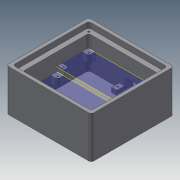
# Autodesk Inventor part: Part1
Saved by Autodesk Inventor 2014 SP1 (Build 180222100, 222)
## iProperties
Created: 2015-04-01
Part Number: Part1
Material: Generic
Document SubType Name: Modeling
Designer: tom
Density: 1 g/cm^3
Appearance: Default
Author: tom
Autodesk Inventor part; units mm, degrees
note: some values were not read from the file. Chosen so that the rebuilt part matches the saved one: sketch regions of "Extrusion8".
ref_plane "YZ Plane" through (0, 0, 0) normal (1, 0, 0) x (0, 1, 0)
ref_plane "XZ Plane" through (0, 0, 0) normal (0, 1, 0) x (-1, 0, 0)
ref_plane "XY Plane" through (0, 0, 0) normal (0, 0, 1) x (1, 0, 0)
sketch "Sketch1" plane through (0, 0, 0) normal (0, 1, 0) x (-1, 0, 0)
  line L0 (80.9542, -63.5193) -> (-4.7708, -63.5193)
  line L1 (-4.7708, -63.5193) -> (-4.7708, 19.0307)
  line L2 (-4.7708, 19.0307) -> (80.9542, 19.0307)
  line L3 (80.9542, 19.0307) -> (80.9542, -63.5193)
  line L4 (-14.7708, -73.5193) -> (90.9542, -73.5193)
  line L5 (90.9542, -73.5193) -> (90.9542, 29.0307)
  line L6 (90.9542, 29.0307) -> (-14.7708, 29.0307)
  line L7 (-14.7708, 29.0307) -> (-14.7708, -73.5193)
  point P0 (0, 0)
  dimension "d0" = 85.725
  dimension "d1" = 82.55
  dimension "d2" = 10
  constraints: 16 end point, 4 parallel, 2 perpendicular, 1 horizontal, 3 other
  measures "d0" distance of L0.start L0.end
  measures "d1" distance of L0.end L1.end
  measures "d2" distance between parallel lines of L3 L5
extrude "Extrusion1" add sketch "Sketch1" along normal blind 5 contours L0 L1 L2 L3 | L7 L6 L5 L4
sketch "Sketch2" plane through (0, 5, 0) normal (0, 1, 0) x (1, 0, 0)
  line L0 (14.7708, 73.5193) -> (-90.9542, 73.5193) projected
  line L1 (-90.9542, 73.5193) -> (-90.9542, -29.0307) projected
  line L2 (-90.9542, -29.0307) -> (14.7708, -29.0307) projected
  line L3 (14.7708, -29.0307) -> (14.7708, 73.5193) projected
  line L4 (-80.9542, 63.5193) -> (4.7708, 63.5193)
  line L5 (4.7708, 63.5193) -> (4.7708, -19.0307)
  line L6 (4.7708, -19.0307) -> (-80.9542, -19.0307)
  line L7 (-80.9542, -19.0307) -> (-80.9542, 63.5193)
  point P0 (0, 0)
  dimension "d5" = 85.725
  dimension "d6" = 82.55
  dimension "d7" = 10
  dimension "d8" = 10
  constraints: 8 end point, 3 perpendicular, 1 parallel
  measures "d5" distance of L4.start L4.end
  measures "d6" distance of L4.end L5.end
  measures "d7" distance between parallel lines of L1 L7
  measures "d8" distance between parallel lines of L0 L4
extrude "Extrusion2" add sketch "Sketch2" along normal blind 40
fillet "Fillet1" radius 3.175 8 edges at (-80.9542, 25, -63.5193) (4.7708, 25, -63.5193) (-80.9542, 25, 19.0307) (4.7708, 25, 19.0307) (-90.9542, 22.5, -73.5193) (14.7708, 22.5, -73.5193) (-90.9542, 22.5, 29.0307) (14.7708, 22.5, 29.0307)
sketch "Sketch3" plane through (11.5958, 0, -73.5193) normal (0, 0, -1) x (-1, 0, 0)
  line L0 (10, 5) -> (89.375, 5) projected
  circle A0 centre (25.875, 8.175) radius 2.3813
  circle A1 centre (35.4, 8.175) radius 2.3812
  circle A2 centre (44.925, 8.175) radius 2.3812
  circle A3 centre (25.875, 17.7) radius 2.3812
  circle A4 centre (44.925, 17.7) radius 2.3812
  line L1 (6.825, 45) -> (6.825, 5) projected
  line L2 (25.875, 20.0813) -> (44.925, 20.0813)
  line L3 (47.3062, 17.7) -> (47.3062, 8.175)
  line L4 (44.925, 5.7938) -> (25.875, 5.7937)
  line L5 (23.4937, 8.175) -> (23.4937, 17.7)
  point P0 (11.5958, 0)
  dimension "d12" = 4.7625
  dimension "d13" = 4.7625
  dimension "d14" = 4.7625
  dimension "d15" = 9.525
  dimension "d16" = 9.525
  dimension "d17" = 3.175
  dimension "d18" = 4.7625
  dimension "d19" = 4.7625
  dimension "d20" = 9.525
  dimension "d21" = 9.525
  dimension "d22" = 19.05
  dimension "d23" = 19.05
  constraints: 8 end point, 8 point on circle, 5 centre point, 5 tangent, 2 perpendicular
  measures "d12" diameter of A0
  measures "d13" diameter of A1
  measures "d14" diameter of A2
  measures "d15" distance of A0.centre A1.centre
  measures "d16" distance of A2.centre A1.centre
  measures "d17" distance from line of L0 A0.centre
  measures "d18" diameter of A3
  measures "d19" diameter of A4
  measures "d20" distance of A0.centre A3.centre
  measures "d21" distance of A4.centre A2.centre
  measures "d22" distance from line of L1 A0.centre
  measures "d23" distance of A4.centre A3.centre
extrude "Extrusion3" cut sketch "Sketch3" against normal blind 10 contours A0 | A1 | A0 L5 A3 L2 A4 L3 A2 L4 | A3 | A2 | A4
sketch "Sketch4" plane through (-77.7792, 5, -63.5193) normal (0, 0, 1) x (1, 0, 0)
  arc A0 (63.5, 0.7937) -> (65.8813, 3.175) centre (63.5, 3.175) ccw projected
  line L0 (63.5, 0.7937) -> (44.45, 0.7938) projected
  arc A1 (42.0688, 3.175) -> (44.45, 0.7938) centre (44.45, 3.175) ccw projected
  line L1 (79.375, 40) -> (79.375, 0) projected
  line L2 (79.375, 0) -> (0, 0) projected
  circle A2 centre (44.45, 3.175) radius 2.3812
  circle A3 centre (63.5, 3.175) radius 2.3813
  circle A4 centre (53.975, 3.175) radius 2.3812
  line L3 (46.8313, 3.175) -> (47.698, 5.5563)
  line L4 (46.8313, 3.175) -> (49.3653, 3.175) construction
  line L5 (51.5938, 3.175) -> (50.727, 5.5563)
  line L6 (51.5938, 3.175) -> (54.1278, 3.175) construction
  line L7 (50.727, 5.5563) -> (47.698, 5.5563)
  line L8 (56.3563, 3.175) -> (57.223, 5.5563)
  line L9 (61.1188, 3.175) -> (60.252, 5.5563)
  line L10 (60.252, 5.5563) -> (57.223, 5.5563)
  line L11 (42.0688, 3.175) -> (41.202, 5.5563)
  line L12 (41.202, 5.5563) -> (34.852, 5.5563)
  line L13 (34.852, 5.5563) -> (34.852, 0)
  line L14 (65.8813, 3.175) -> (66.748, 5.5562)
  line L15 (66.748, 5.5562) -> (73.098, 5.5562)
  line L16 (0, 0) -> (0, 40) projected
  line L17 (73.098, 5.5562) -> (73.098, 0)
  point P0 (77.7792, -5)
  dimension "d26" = 70
  dimension "d27" = 110
  dimension "d28" = 6.35
  dimension "d31" = 6.35
  constraints: 28 end point, 6 parallel, 6 point on circle, 3 centre point, 2 coincident, 2 collinear, 2 equal length, 2 horizontal, 2 perpendicular, 2 point on line
  measures "d26" angle of L4 L3
  measures "d27" angle of L6 L5
  measures "d28" distance of L11.end L12.end
  measures "d31" distance of L14.end L15.end
extrude "Extrusion4" add sketch "Sketch4" along normal blind 9.525 contours A0 L14 L15 L17 L2 L13 L12 L11 A1 L0 | L0 A4 L8 L10 L9 A3 | L0 A2 L3 L7 L5 A4
ref_plane "Work Plane1" through (-40.0917, 29.5, -24.6568) normal (0, -1, 0) x (1, 0, 0)
sketch "Sketch6" plane through (0, 45, 0) normal (0, 1, 0) x (1, 0, 0)
  arc A0 (11.5958, -29.0307) -> (14.7708, -25.8557) centre (11.5958, -25.8557) ccw projected
  line L0 (14.7708, -25.8557) -> (14.7708, 70.3443) projected
  arc A1 (14.7708, 70.3443) -> (11.5958, 73.5193) centre (11.5958, 70.3443) ccw projected
  line L1 (11.5958, 73.5193) -> (-87.7792, 73.5193) projected
  arc A2 (-87.7792, 73.5193) -> (-90.9542, 70.3443) centre (-87.7792, 70.3443) ccw projected
  line L2 (-90.9542, 70.3443) -> (-90.9542, -25.8557) projected
  arc A3 (-90.9542, -25.8557) -> (-87.7792, -29.0307) centre (-87.7792, -25.8557) ccw projected
  line L3 (-87.7792, -29.0307) -> (11.5958, -29.0307) projected
  line L4 (-86.9542, 69.5193) -> (10.7708, 69.5193)
  line L5 (10.7708, 69.5193) -> (10.7708, -25.0307)
  line L6 (10.7708, -25.0307) -> (-86.9542, -25.0307)
  line L7 (-86.9542, -25.0307) -> (-86.9542, 69.5193)
  point P0 (0, 0)
  dimension "d38" = 4
  dimension "d39" = 4
  dimension "d40" = 4
  dimension "d41" = 4
  constraints: 8 end point, 2 parallel, 1 horizontal, 1 perpendicular
  measures "d38" distance between parallel lines of L1 L4
  measures "d39" distance between parallel lines of L2 L7
  measures "d40" distance between parallel lines of L3 L6
  measures "d41" distance between parallel lines of L0 L5
extrude "Extrusion6" add sketch "Sketch6" along normal blind 7
fillet "Fillet2" radius 3.175 4 edges at (10.7708, 48.5, -69.5193) (-86.9542, 48.5, -69.5193) (-86.9542, 48.5, 25.0307) (10.7708, 48.5, 25.0307)
sketch "Sketch7" plane through (0, 45, 0) normal (0, 1, 0) x (1, 0, 0)
  line L0 (7.5958, 69.5193) -> (-83.7792, 69.5193) projected
  line L1 (4.7708, 60.3443) -> (4.7708, -15.8557) projected
  line L2 (1.5958, -19.0307) -> (-77.7792, -19.0307) projected
  line L3 (-80.9542, -15.8557) -> (-80.9542, 60.3443) projected
  arc A0 (-77.7792, 63.5193) -> (-80.9542, 60.3443) centre (-77.7792, 60.3443) ccw projected
  line L4 (-38.0917, 69.5193) -> (-38.0917, -19.0307) construction
  line L5 (-80.9542, 22.2443) -> (4.7708, 22.2443) construction
  line L6 (-77.7792, 60.3443) -> (-82.7289, 65.2941) construction
  circle A1 centre (-82.7289, 65.2941) radius 1.27
  circle A2 centre (6.5456, 65.2941) radius 1.27
  circle A3 centre (-82.7289, -20.8054) radius 1.27
  circle A4 centre (6.5456, -20.8054) radius 1.27
  point P0 (0, 0)
  dimension "d44" = 7
  dimension "d45" = 2.54
  constraints: 6 end point, 4 centre point, 4 midpoint, 3 symmetric about line, 1 coincident, 3 other
  measures "d44" distance of L6.start L6.end
  measures "d45" diameter of A1
extrude "Extrusion7" cut sketch "Sketch7" against normal blind 12.7
sketch "Sketch8" plane through (-40.0917, 29.5, -24.6568) normal (0, -1, 0) x (1, 0, 0)
  circle A0 centre (39.5, -2.5) radius 1 projected
  circle A1 centre (39.5, -33.5) radius 1 projected
  circle A2 centre (-35.5, -2.5) radius 1 projected
  circle A3 centre (-35.5, -33.5) radius 1 projected
  line L0 (-38, 0) -> (42, 0) projected
  line L1 (-38, -36) -> (-38, 0) projected
  line L2 (42, -36) -> (-38, -36) projected
  line L3 (42, 0) -> (42, -36) projected
  arc A4 (39.5, -30.5) -> (36.5, -33.5) centre (39.5, -33.5) ccw
  circle A5 centre (-42.6372, 45.4622) radius 1.27 projected
  circle A6 centre (-42.6372, -40.6372) radius 1.27 projected
  circle A7 centre (46.6372, -40.6372) radius 1.27 projected
  circle A8 centre (46.6372, 45.4622) radius 1.27 projected
  arc A9 (50.8625, 46.5125) -> (47.6875, 49.6875) centre (47.6875, 46.5125) ccw projected
  line L4 (50.8625, 46.5125) -> (50.8625, -41.6875) projected
  arc A10 (47.6875, -44.8625) -> (50.8625, -41.6875) centre (47.6875, -41.6875) ccw projected
  line L5 (47.6875, -44.8625) -> (-43.6875, -44.8625) projected
  arc A11 (-46.8625, -41.6875) -> (-43.6875, -44.8625) centre (-43.6875, -41.6875) ccw projected
  line L6 (-46.8625, -41.6875) -> (-46.8625, 46.5125) projected
  arc A12 (-43.6875, 49.6875) -> (-46.8625, 46.5125) centre (-43.6875, 46.5125) ccw projected
  line L7 (-43.6875, 49.6875) -> (47.6875, 49.6875) projected
  line L8 (44.8625, -35.6875) -> (44.8625, 40.5125) projected
  arc A13 (44.8625, 40.5125) -> (41.6875, 43.6875) centre (41.6875, 40.5125) ccw projected
  line L9 (41.6875, 43.6875) -> (-37.6875, 43.6875) projected
  arc A14 (-37.6875, 43.6875) -> (-40.8625, 40.5125) centre (-37.6875, 40.5125) ccw projected
  line L10 (-40.8625, 40.5125) -> (-40.8625, -35.6875) projected
  arc A15 (-40.8625, -35.6875) -> (-37.6875, -38.8625) centre (-37.6875, -35.6875) ccw projected
  line L11 (-37.6875, -38.8625) -> (41.6875, -38.8625) projected
  arc A16 (41.6875, -38.8625) -> (44.8625, -35.6875) centre (41.6875, -35.6875) ccw projected
  line L12 (36.5, -33.5) -> (36.5, -38.8625)
  line L13 (39.5, -30.5) -> (44.8625, -30.5)
  line L14 (2, -44.8625) -> (2, 5.6581) construction
  line L15 (42, -18) -> (-38, -18) construction
  circle A17 centre (39.5, -33.5) radius 0.762
  arc A18 (-32.5, -33.5) -> (-35.5, -30.5) centre (-35.5, -33.5) ccw
  line L16 (-32.5, -33.5) -> (-32.5, -38.8625)
  line L17 (-35.5, -30.5) -> (-40.8625, -30.5)
  circle A19 centre (-35.5, -33.5) radius 0.762
  arc A20 (36.5, -2.5) -> (39.5, -5.5) centre (39.5, -2.5) ccw
  line L18 (39.5, -5.5) -> (44.8625, -5.5)
  circle A21 centre (39.5, -2.5) radius 0.762
  line L19 (36.5, -2.5) -> (36.5, 0)
  line L20 (36.5, 0) -> (44.8625, 0)
  line L21 (-35.5, -5.5) -> (-40.8625, -5.5)
  arc A22 (-35.5, -5.5) -> (-32.5, -2.5) centre (-35.5, -2.5) ccw
  circle A23 centre (-35.5, -2.5) radius 0.762
  line L22 (-32.5, -2.5) -> (-32.5, 0)
  line L23 (-32.5, 0) -> (-40.8625, 0)
  arc A24 (41.6875, -38.8625) -> (44.8625, -35.6875) centre (41.6875, -35.6875) ccw
  line L24 (-40.8625, -30.5) -> (-40.8625, -35.6875)
  line L25 (-37.6875, -38.8625) -> (-32.5, -38.8625)
  line L26 (36.5, -38.8625) -> (41.6875, -38.8625)
  line L27 (44.8625, -30.5) -> (44.8625, -35.6875)
  arc A25 (-40.8625, -35.6875) -> (-37.6875, -38.8625) centre (-37.6875, -35.6875) ccw
  line L28 (-40.8625, 0) -> (-40.8625, -5.5)
  line L29 (44.8625, 0) -> (44.8625, -5.5)
  point P0 (40.0917, 24.6568)
  dimension "d49" = 1.524
  constraints: 38 end point, 18 symmetric about line, 12 point on circle, 10 centre point, 10 point on line, 8 tangent, 7 coincident, 6 perpendicular, 3 midpoint, 2 collinear, 1 parallel, 6 other
  measures "d49" diameter of A17
extrude "Extrusion8" add sketch "Sketch8" along normal blind 9.525 contours A0 | A1 | A2 | A3 | L0 L22 A22 L21 L1 | L1 L21 L10 L23 | L0 L3 L18 A20 L19 | L17 A18 L16 L2 L1 | L1 L2 L16 L11 A15 L10 L17 | L20 L8 L18 L3 | L13 L8 A16 L11 L12 L2 L3 | L3 L2 L12 A4 L13
sketch "Sketch9" plane through (-40.0917, 29.5, -24.6568) normal (0, 1, 0) x (1, 0, 0)
  arc A0 (-35.5, 30.5) -> (-32.5, 33.5) centre (-35.5, 33.5) ccw projected
  line L0 (-40.8625, 0) -> (-40.8625, 5.5) projected
  line L1 (-32.5, 0) -> (-40.8625, 0) projected
  line L2 (-32.5, 2.5) -> (-32.5, 0) projected
  arc A1 (-32.5, 2.5) -> (-35.5, 5.5) centre (-35.5, 2.5) ccw projected
  line L3 (-40.8625, 5.5) -> (-35.5, 5.5) projected
  line L4 (36.5, 0) -> (36.5, 2.5) projected
  line L5 (44.8625, 0) -> (36.5, 0) projected
  line L6 (44.8625, 5.5) -> (44.8625, 0) projected
  line L7 (39.5, 5.5) -> (44.8625, 5.5) projected
  arc A2 (39.5, 5.5) -> (36.5, 2.5) centre (39.5, 2.5) ccw projected
  circle A3 centre (-35.5, 33.5) radius 0.762
  circle A4 centre (-35.5, 2.5) radius 0.762
  circle A5 centre (39.5, 2.5) radius 0.762
  point P0 (40.0917, -24.6568)
  dimension "d52" = 1.524
  dimension "d53" = 1.524
  dimension "d54" = 1.524
  constraints: 3 centre point, 3 coincident
  measures "d52" diameter of A3
  measures "d53" diameter of A4
  measures "d54" diameter of A5
extrude "Extrusion9" cut sketch "Sketch9" against normal blind 12.7 contours A3 | A4 | A5
ref_plane "Work Plane2" through (1.9083, 23.4125, -21.8318) normal (0, -1, 0) x (1, 0, 0)
sketch "Sketch10" plane through (1.9083, 23.4125, -21.8318) normal (0, -1, 0) x (1, 0, 0)
  circle A0 centre (-77.5, 2.5) radius 3
  circle A1 centre (-2.5, 2.5) radius 3
  circle A2 centre (-2.5, 35.5) radius 3
  circle A3 centre (-77.5, 35.5) radius 3
  line L0 (-74.5, 2.5) -> (-74.5, -2.8589)
  circle A4 centre (-84.6372, 42.6372) radius 1.27 projected
  circle A5 centre (-84.6372, -43.4622) radius 1.27 projected
  circle A6 centre (4.6372, -43.4622) radius 1.27 projected
  circle A7 centre (4.6372, 42.6372) radius 1.27 projected
  arc A8 (8.8625, 43.6875) -> (5.6875, 46.8625) centre (5.6875, 43.6875) ccw projected
  line L1 (8.8625, 43.6875) -> (8.8625, -44.5125) projected
  arc A9 (5.6875, -47.6875) -> (8.8625, -44.5125) centre (5.6875, -44.5125) ccw projected
  line L2 (5.6875, -47.6875) -> (-85.6875, -47.6875) projected
  arc A10 (-88.8625, -44.5125) -> (-85.6875, -47.6875) centre (-85.6875, -44.5125) ccw projected
  line L3 (-88.8625, -44.5125) -> (-88.8625, 43.6875) projected
  arc A11 (-85.6875, 46.8625) -> (-88.8625, 43.6875) centre (-85.6875, 43.6875) ccw projected
  line L4 (-85.6875, 46.8625) -> (5.6875, 46.8625) projected
  line L5 (2.8625, -38.5125) -> (2.8625, 37.6875) projected
  arc A12 (2.8625, 37.6875) -> (-0.3125, 40.8625) centre (-0.3125, 37.6875) ccw projected
  line L6 (-0.3125, 40.8625) -> (-79.6875, 40.8625) projected
  arc A13 (-79.6875, 40.8625) -> (-82.8625, 37.6875) centre (-79.6875, 37.6875) ccw projected
  line L7 (-82.8625, 37.6875) -> (-82.8625, -38.5125) projected
  arc A14 (-82.8625, -38.5125) -> (-79.6875, -41.6875) centre (-79.6875, -38.5125) ccw projected
  line L8 (-79.6875, -41.6875) -> (-0.3125, -41.6875) projected
  arc A15 (-0.3125, -41.6875) -> (2.8625, -38.5125) centre (-0.3125, -38.5125) ccw projected
  line L9 (-74.5, -2.8589) -> (-82.8625, -2.8589)
  line L10 (-77.5, 5.5) -> (-82.8625, 5.5)
  line L11 (-82.8625, -2.8589) -> (-82.8625, 5.5)
  line L12 (-77.5, 32.5) -> (-82.8625, 32.5)
  line L13 (-74.5, 35.5) -> (-74.5, 40.8625)
  line L14 (-2.5, 32.5) -> (2.8625, 32.5)
  line L15 (-2.5, 5.5) -> (2.8625, 5.5)
  line L16 (-5.5, 2.5) -> (-5.5, -2.8589)
  line L17 (-5.5, -2.8589) -> (2.8625, -2.8589)
  line L18 (2.8625, -2.8589) -> (2.8625, 5.5)
  line L19 (-5.5, 35.5) -> (-5.5, 40.8625)
  circle A16 centre (-77.5, 2.5) radius 0.762
  circle A17 centre (-2.5, 2.5) radius 0.762
  circle A18 centre (-2.5, 35.5) radius 0.762
  circle A19 centre (-77.5, 35.5) radius 0.762
  point P0 (-1.9083, 21.8318)
  dimension "d57" = 6
  dimension "d58" = 6
  dimension "d59" = 6
  dimension "d60" = 6
  dimension "d63" = 1.524
  dimension "d64" = 1.524
  dimension "d65" = 1.524
  dimension "d66" = 1.524
  constraints: 24 end point, 9 perpendicular, 8 centre point, 8 point on circle, 8 point on line, 8 tangent, 4 coincident, 1 collinear, 1 parallel
  measures "d57" diameter of A0
  measures "d58" diameter of A1
  measures "d59" diameter of A2
  measures "d60" diameter of A3
  measures "d63" diameter of A16
  measures "d64" diameter of A17
  measures "d65" diameter of A18
  measures "d66" diameter of A19
extrude "Extrusion10" add sketch "Sketch10" along normal blind 9.525 contours A0 | L0 L9 L7 L10 A0 | L7 A13 L6 L13 A3 L12 | A3 | L6 A12 L5 L14 A2 L19 | L17 L16 A1 L15 L5 | A2 | A1
sketch "Sketch11" plane through (-42.9271, 10.5563, -63.5193) normal (0, 1, 0) x (1, 0, 0)
  circle A0 centre (3.175, -4.7625) radius 1.524 projected
  circle A1 centre (35.0709, -4.7625) radius 1.524 projected
  circle A2 centre (3.175, -4.7625) radius 0.762
  circle A3 centre (35.0709, -4.7625) radius 0.762
  point P0 (42.9271, -63.5193)
  dimension "d67" = 1.524
  dimension "d68" = 1.524
  constraints: 2 centre point, 2 coincident
  measures "d67" diameter of A2
  measures "d68" diameter of A3
extrude "Extrusion11" cut sketch "Sketch11" against normal blind 8 contours A2 | A3
sketch "Sketch12" plane through (7.5958, 45, 25.0307) normal (0, 0, -1) x (-1, 0, 0)
  line L0 (91.375, 0) -> (0, 0) projected
  line L1 (0, 7) -> (91.375, 7) projected
  line L2 (45.6875, 7) -> (45.6875, 0) construction
  line L3 (42.1875, 7) -> (42.1875, 0)
  line L4 (49.1875, 7) -> (49.1875, 0)
  line L5 (42.1875, 5.5) -> (49.1875, 5.5)
  line L6 (42.1875, 0) -> (42.1875, -3)
  line L7 (42.1875, -3) -> (49.1875, -3)
  line L8 (49.1875, -3) -> (49.1875, 0)
  point P0 (7.5958, -45)
  dimension "d71" = 7
  dimension "d72" = 3.5
  dimension "d73" = 5.5
  dimension "d74" = 3
  constraints: 14 end point, 6 point on line, 4 perpendicular, 2 midpoint, 2 parallel
  measures "d71" distance between parallel lines of L4 L3
  measures "d72" distance between parallel lines of L2 L3
  measures "d73" distance between parallel lines of L0 L5
  measures "d74" distance of L3.end L6.end
extrude "Extrusion12" cut sketch "Sketch12" against normal blind 2 contours L8 L7 L6 L0 | L0 L3 L5 L4
sketch "Sketch13" plane through (1.5958, 5, 19.0307) normal (0, 0, -1) x (-1, 0, 0)
  line L0 (79.375, 0) -> (0, 0) projected
  line L1 (36.1875, 37) -> (36.1875, 45.5) projected
  line L2 (43.1875, 37) -> (36.1875, 37) projected
  line L3 (43.1875, 45.5) -> (43.1875, 37) projected
  line L4 (36.1875, 45.5) -> (43.1875, 45.5) projected
  line L5 (38.1875, 37) -> (38.1875, 0)
  line L6 (41.1875, 37) -> (41.1875, 0)
  line L7 (39.6875, 37) -> (39.6875, 0) construction
  point P0 (1.5958, -5)
  dimension "d77" = 3
  dimension "d78" = 1.5
  constraints: 6 end point, 4 point on line, 2 midpoint, 2 perpendicular
  measures "d77" distance between parallel lines of L5 L6
  measures "d78" distance between parallel lines of L7 L6
extrude "Extrusion13" cut sketch "Sketch13" against normal blind 6
equation "\"d8\" = d7"
equation "\"d16\" = d15"
equation "\"d21\" = d20"
equation "\"d39\" = d38"
equation "\"d40\" = d39"
equation "\"d41\" = d38"
equation "\"d53\" = d52"
equation "\"d54\" = d52"
equation "\"d72\" = 0.5 * d71"
equation "\"d78\" = 0.5 * d77"
body "Solid1"
